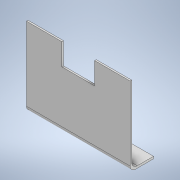
# Autodesk Inventor part: płyta_dla_arduino
Saved by Autodesk Inventor 2021 (Build 250183000, 183)
## iProperties
Created: 2022-02-05
Part Number: płyta_dla_arduino
Material: Generic
Document SubType Name: Modeling
Designer: Łukasz
Density: 1 g/cm^3
Appearance: Default
Author: Łukasz
Autodesk Inventor part; units mm, degrees
ref_plane "YZ Plane" through (0, 0, 0) normal (1, 0, 0) x (0, 1, 0)
ref_plane "XZ Plane" through (0, 0, 0) normal (0, 1, 0) x (-1, 0, 0)
ref_plane "XY Plane" through (0, 0, 0) normal (0, 0, 1) x (1, 0, 0)
sketch "Sketch1" plane through (0, 0, 0) normal (0, 0, 1) x (1, 0, 0)
  line L0 (-15.6474, 9.6574) -> (174.3526, 9.6574)
  line L1 (174.3526, 9.6574) -> (174.3526, -135.3426)
  line L2 (174.3526, -135.3426) -> (-15.6474, -135.3426)
  line L3 (-15.6474, -135.3426) -> (-15.6474, 9.6574)
  line L4 (49.3526, 9.6574) -> (109.3526, 9.6574)
  line L5 (109.3526, 9.6574) -> (109.3526, -30.3426)
  line L6 (109.3526, -30.3426) -> (49.3526, -30.3426)
  line L7 (49.3526, -30.3426) -> (49.3526, 9.6574)
  point P0 (0, 0)
  dimension "d0" = 190
  dimension "d1" = 145
  dimension "d2" = 60
  dimension "d3" = 40
  dimension "d4" = 65
  constraints: 16 end point, 4 parallel, 2 horizontal, 2 perpendicular, 1 point on line
  measures "d0" distance of L1.end L2.end
  measures "d1" distance of L0.end L1.end
  measures "d2" distance of L5.end L6.end
  measures "d3" distance of L4.end L5.end
  measures "d4" distance between parallel lines of L3 L7
extrude "Extrusion1" add sketch "Sketch1" along normal blind 3 contours L0 L7 L6 L5 L1 L2 L3
sketch "Sketch2" plane through (0, 0, 0) normal (0, 0, -1) x (-1, 0, 0)
  line L0 (15.6474, -135.3426) -> (-174.3526, -135.3426) projected
  line L1 (-174.3526, -135.3426) -> (-174.3526, 9.6574) projected
  line L2 (15.6474, -135.3426) -> (-174.3526, -135.3426)
  line L3 (-174.3526, -135.3426) -> (-174.3526, -131.3426)
  line L4 (-174.3526, -131.3426) -> (15.6474, -131.3426)
  line L5 (15.6474, -131.3426) -> (15.6474, -135.3426)
  point P0 (0, 0)
  dimension "d7" = 4
  constraints: 8 end point, 2 parallel, 1 horizontal, 1 perpendicular, 1 point on line
  measures "d7" distance of L2.end L3.end
extrude "Extrusion2" add sketch "Sketch2" along normal blind 40
fillet "Fillet1" radius 10 2 edges at (79.3526, -131.3426, 0) (79.3526, -135.3426, 3)
body "Solid1"
